Autodesk Fusion 360 part; units mm, degrees
(part 2 of 2)
  spline S14 degree 5 poles (-13.964533, 25.2) (-13.962061, 24.966553) (-13.956383, 24.502635) (-13.94566, 23.815681) (-13.926878, 22.917891) (-13.895401, 21.828032) (-13.855137, 20.773732) (-13.80525, 19.758375) (-13.745091, 18.78459) (-13.674758, 17.851981) (-13.594892, 16.957952) (-13.523933, 16.271322) (-13.466984, 15.771448) (-13.427386, 15.444802) (-13.407179, 15.28313) knots 0 0 0 0 0 0 0.1 0.2 0.3 0.4 0.5 0.6 0.7 0.8 0.9 1 1 1 1 1 1
  spline S15 degree 5 poles (-13.407179, 15.28313) (-13.396137, 15.263359) (-13.378996, 15.22331) (-13.368109, 15.161714) (-13.383287, 15.076541) (-13.451281, 14.964449) (-13.566539, 14.845147) (-13.725152, 14.715443) (-13.922038, 14.571096) (-14.152128, 14.407493) (-14.411349, 14.220248) (-14.697981, 14.00591) (-15.0128, 13.762359) (-15.357694, 13.488824) (-15.73468, 13.186004) (-16.144739, 12.856162) (-16.586746, 12.503236) (-17.056304, 12.132966) (-17.54468, 11.753005) (-18.03747, 11.373112) (-18.516745, 11.004243) (-18.963466, 10.657557) (-19.359795, 10.343456) (-19.691437, 10.070608) (-19.950048, 9.844948) (-20.135514, 9.668721) (-20.258658, 9.539357) (-20.342872, 9.448765) (-20.41611, 9.386384) (-20.504485, 9.341635) (-20.623844, 9.307073) (-20.78081, 9.278288) (-20.976661, 9.252807) (-21.210563, 9.229259) (-21.482071, 9.206674) (-21.790708, 9.184492) (-22.067067, 9.166839) (-22.290806, 9.15361) (-22.447275, 9.144795) (-22.527337, 9.140389) knots 0 0 0 0 0 0 0.02857143 0.05714286 0.08571429 0.11428571 0.14285714 0.17142857 0.2 0.22857143 0.25714286 0.28571429 0.31428571 0.34285714 0.37142857 0.4 0.42857143 0.45714286 0.48571429 0.51428571 0.54285714 0.57142857 0.6 0.62857143 0.65714286 0.68571429 0.71428571 0.74285714 0.77142857 0.8 0.82857143 0.85714286 0.88571429 0.91428571 0.94285714 0.97142857 1 1 1 1 1 1
  spline S16 degree 5 poles (-22.527337, 9.140389) (-22.534782, 9.132257) (-22.551108, 9.119693) (-22.579895, 9.111944) (-22.626933, 9.123822) (-22.704194, 9.176034) (-22.81318, 9.266751) (-22.971739, 9.396826) (-23.195327, 9.565352) (-23.491204, 9.768427) (-23.851155, 9.997537) (-24.255113, 10.24102) (-24.676282, 10.485947) (-25.085787, 10.719892) (-25.45738, 10.932679) (-25.772439, 11.118288) (-26.024118, 11.276365) (-26.223686, 11.414734) (-26.399129, 11.548396) (-26.585024, 11.694604) (-26.814317, 11.868763) (-27.110137, 12.080424) (-27.475633, 12.328182) (-27.891521, 12.598759) (-28.3256, 12.872564) (-28.739447, 13.127746) (-29.096109, 13.344754) (-29.367661, 13.510891) (-29.542161, 13.624396) (-29.632469, 13.699901) (-29.679781, 13.770002) (-29.730096, 13.86743) (-29.810663, 14.006795) (-29.915111, 14.173854) (-30.022328, 14.343768) (-30.107951, 14.492643) (-30.162056, 14.615407) (-30.190972, 14.726246) (-30.207343, 14.846076) (-30.222219, 14.991915) (-30.24042, 15.171174) (-30.263532, 15.386409) (-30.290852, 15.637231) (-30.321406, 15.923867) (-30.354419, 16.247692) (-30.389152, 16.610252) (-30.424903, 17.012708) (-30.460944, 17.455117) (-30.496481, 17.935767) (-30.530614, 18.450516) (-30.562281, 18.992027) (-30.590316, 19.550497) (-30.613514, 20.114573) (-30.630694, 20.672199) (-30.640764, 21.211485) (-30.642783, 21.721575) (-30.636028, 22.193507) (-30.620056, 22.621096) (-30.594767, 23.001764) (-30.560482, 23.337543) (-30.517829, 23.633921) (-30.46762, 23.898494) (-30.410725, 24.139655) (-30.347958, 24.365361) (-30.279935, 24.581643) (-30.207018, 24.791997) (-30.144919, 24.956973) (-30.096257, 25.079107) (-30.062889, 25.15982) (-30.045972, 25.2) knots 0 0 0 0 0 0 0.01538462 0.03076923 0.04615385 0.06153846 0.07692308 0.09230769 0.10769231 0.12307692 0.13846154 0.15384615 0.16923077 0.18461538 0.2 0.21538462 0.23076923 0.24615385 0.26153846 0.27692308 0.29230769 0.30769231 0.32307692 0.33846154 0.35384615 0.36923077 0.38461538 0.4 0.41538462 0.43076923 0.44615385 0.46153846 0.47692308 0.49230769 0.50769231 0.52307692 0.53846154 0.55384615 0.56923077 0.58461538 0.6 0.61538462 0.63076923 0.64615385 0.66153846 0.67692308 0.69230769 0.70769231 0.72307692 0.73846154 0.75384615 0.76923077 0.78461538 0.8 0.81538462 0.83076923 0.84615385 0.86153846 0.87692308 0.89230769 0.90769231 0.92307692 0.93846154 0.95384615 0.96923077 0.98461538 1 1 1 1 1 1
  spline S17 degree 5 poles (-35.799999, 25.2) (-35.857716, 25.156712) (-35.97592, 25.068059) (-36.161536, 24.928847) (-36.425914, 24.730563) (-36.786328, 24.460253) (-37.178908, 24.165818) (-37.605546, 23.845839) (-38.06599, 23.500506) (-38.557778, 23.131666) (-39.078002, 22.741497) (-39.514822, 22.413883) (-39.853268, 22.160048) (-40.083634, 21.987274) (-40.2, 21.9) knots 0 0 0 0 0 0 0.1 0.2 0.3 0.4 0.5 0.6 0.7 0.8 0.9 1 1 1 1 1 1
  spline S18 degree 5 poles (-7.251685, 9.474688) (-7.316766, 9.512048) (-7.450091, 9.589871) (-7.660018, 9.71659) (-7.959502, 9.906733) (-8.357963, 10.176766) (-8.767002, 10.471566) (-9.170812, 10.780262) (-9.554132, 11.090061) (-9.904845, 11.387591) (-10.217116, 11.660275) (-10.492886, 11.897621) (-10.739118, 12.09218) (-10.96578, 12.240707) (-11.183637, 12.344934) (-11.401893, 12.413255) (-11.626685, 12.459399) (-11.860987, 12.495777) (-12.104321, 12.528522) (-12.35221, 12.550684) (-12.59883, 12.547293) (-12.840058, 12.502059) (-13.076714, 12.403991) (-13.316787, 12.252645) (-13.5718, 12.05426) (-13.853764, 11.818935) (-14.172187, 11.557638) (-14.530366, 11.278714) (-14.92494, 10.987016) (-15.348078, 10.685204) (-15.788916, 10.374414) (-16.23528, 10.055179) (-16.67533, 9.728263) (-17.099141, 9.395474) (-17.500548, 9.060643) (-17.878143, 8.730033) (-18.23344, 8.410834) (-18.569489, 8.109951) (-18.889355, 7.832721) (-19.194554, 7.581563) (-19.483748, 7.354873) (-19.750714, 7.145276) (-19.985619, 6.940757) (-20.178259, 6.727494) (-20.32065, 6.492138) (-20.409985, 6.224389) (-20.451164, 5.919245) (-20.454223, 5.575435) (-20.432003, 5.194029) (-20.397764, 4.776997) (-20.362746, 4.325755) (-20.333949, 3.839836) (-20.314916, 3.317711) (-20.306339, 2.757479) (-20.306734, 2.157595) (-20.313084, 1.517597) (-20.321495, 0.838812) (-20.327855, 0.125116) (-20.328456, -0.616433) (-20.32074, -1.374637) (-20.303356, -2.134916) (-20.275945, -2.880746) (-20.239009, -3.594886) (-20.193751, -4.260684) (-20.141925, -4.86336) (-20.085669, -5.391269) (-20.027396, -5.837255) (-19.969528, -6.199769) (-19.914629, -6.484576) (-19.863943, -6.704252) (-19.814039, -6.875712) (-19.754645, -7.018248) (-19.664373, -7.151443) (-19.519774, -7.292529) (-19.3074, -7.453568) (-19.035103, -7.638642) (-18.724726, -7.845502) (-18.404345, -8.067303) (-18.100648, -8.294303) (-17.831346, -8.515571) (-17.597303, -8.720715) (-17.387506, -8.901628) (-17.184613, -9.054424) (-16.969919, -9.180947) (-16.729466, -9.291328) (-16.455457, -9.402009) (-16.14484, -9.530988) (-15.798752, -9.69393) (-15.421602, -9.899874) (-15.020326, -10.14724) (-14.603987, -10.426642) (-14.183416, -10.723577) (-13.770811, -11.021141) (-13.379401, -11.302783) (-13.022974, -11.554912) (-12.715738, -11.769892) (-12.471165, -11.94789) (-12.295635, -12.093535) (-12.183275, -12.213403) (-12.10937, -12.312955) (-12.026929, -12.394313) (-11.893759, -12.460455) (-11.701593, -12.520264) (-11.466708, -12.582483) (-11.21561, -12.64913) (-10.970951, -12.706907) (-10.746908, -12.732716) (-10.548658, -12.703423) (-10.36984, -12.605287) (-10.192728, -12.440298) (-9.995867, -12.219618) (-9.759968, -11.95953) (-9.475708, -11.675797) (-9.146515, -11.38075) (-8.783663, -11.084023) (-8.403132, -10.792461) (-8.021772, -10.510367) (-7.653742, -10.2396) (-7.306873, -9.979739) (-6.978942, -9.728205) (-6.660942, -9.481173) (-6.340562, -9.2345) (-6.005554, -8.984635) (-5.647219, -8.729565) (-5.263667, -8.469681) (-4.863667, -8.20886) (-4.463558, -7.952911) (-4.083315, -7.707674) (-3.743007, -7.477316) (-3.458888, -7.262376) (-3.240113, -7.058316) (-3.083992, -6.852825) (-2.978531, -6.629482) (-2.908356, -6.374567) (-2.859179, -6.082202) (-2.823813, -5.761836) (-2.800997, -5.433319) (-2.792171, -5.118206) (-2.799067, -4.832786) (-2.820648, -4.579328) (-2.851306, -4.341342) (-2.883618, -4.0939) (-2.910261, -3.811109) (-2.926583, -3.475921) (-2.931806, -3.084898) (-2.927712, -2.643652) (-2.917854, -2.164229) (-2.906556, -1.661705) (-2.898016, -1.151167) (-2.895328, -0.644408) (-2.89965, -0.147098) (-2.91081, 0.33966) (-2.927794, 0.8181) (-2.94928, 1.292445) (-2.974165, 1.767598) (-3.002065, 2.247839) (-3.033886, 2.735473) (-3.072209, 3.229633) (-3.120043, 3.726674) (-3.179682, 4.220423) (-3.251569, 4.702502) (-3.333056, 5.162573) (-3.417441, 5.588728) (-3.492333, 5.967551) (-3.539956, 6.285114) (-3.546166, 6.532117) (-3.508324, 6.708507) (-3.443506, 6.828224) (-3.396959, 6.924142) (-3.417583, 7.032207) (-3.528131, 7.172298) (-3.728551, 7.349665) (-4.004839, 7.559861) (-4.336561, 7.792682) (-4.700817, 8.034984) (-5.07472, 8.272853) (-5.438381, 8.493996) (-5.777747, 8.690093) (-6.087347, 8.859036) (-6.373518, 9.007565) (-6.650375, 9.148352) (-6.878149, 9.266932) (-7.059607, 9.365713) (-7.186605, 9.437328) (-7.251685, 9.474688) knots 0 0 0 0 0 0 0.00555556 0.01111111 0.01666667 0.02222222 0.02777778 0.03333333 0.03888889 0.04444444 0.05 0.05555556 0.06111111 0.06666667 0.07222222 0.07777778 0.08333333 0.08888889 0.09444444 0.1 0.10555556 0.11111111 0.11666667 0.12222222 0.12777778 0.13333333 0.13888889 0.14444444 0.15 0.15555556 0.16111111 0.16666667 0.17222222 0.17777778 0.18333333 0.18888889 0.19444444 0.2 0.20555556 0.21111111 0.21666667 0.22222222 0.22777778 0.23333333 0.23888889 0.24444444 0.25 0.25555556 0.26111111 0.26666667 0.27222222 0.27777778 0.28333333 0.28888889 0.29444444 0.3 0.30555556 0.31111111 0.31666667 0.32222222 0.32777778 0.33333333 0.33888889 0.34444444 0.35 0.35555556 0.36111111 0.36666667 0.37222222 0.37777778 0.38333333 0.38888889 0.39444444 0.4 0.40555556 0.41111111 0.41666667 0.42222222 0.42777778 0.43333333 0.43888889 0.44444444 0.45 0.45555556 0.46111111 0.46666667 0.47222222 0.47777778 0.48333333 0.48888889 0.49444444 0.5 0.50555556 0.51111111 0.51666667 0.52222222 0.52777778 0.53333333 0.53888889 0.54444444 0.55 0.55555556 0.56111111 0.56666667 0.57222222 0.57777778 0.58333333 0.58888889 0.59444444 0.6 0.60555556 0.61111111 0.61666667 0.62222222 0.62777778 0.63333333 0.63888889 0.64444444 0.65 0.65555556 0.66111111 0.66666667 0.67222222 0.67777778 0.68333333 0.68888889 0.69444444 0.7 0.70555556 0.71111111 0.71666667 0.72222222 0.72777778 0.73333333 0.73888889 0.74444444 0.75 0.75555556 0.76111111 0.76666667 0.77222222 0.77777778 0.78333333 0.78888889 0.79444444 0.8 0.80555556 0.81111111 0.81666667 0.82222222 0.82777778 0.83333333 0.83888889 0.84444444 0.85 0.85555556 0.86111111 0.86666667 0.87222222 0.87777778 0.88333333 0.88888889 0.89444444 0.9 0.90555556 0.91111111 0.91666667 0.92222222 0.92777778 0.93333333 0.93888889 0.94444444 0.95 0.95555556 0.96111111 0.96666667 0.97222222 0.97777778 0.98333333 0.98888889 0.99444444 1 1 1 1 1 1
  spline S19 degree 5 poles (-40.2, 19.435126) (-40.149452, 19.475964) (-40.050433, 19.557248) (-39.90661, 19.679254) (-39.715894, 19.84754) (-39.45302, 20.080899) (-39.140036, 20.348802) (-38.757974, 20.658525) (-38.300256, 21.011032) (-37.779317, 21.398606) (-37.221446, 21.806837) (-36.660563, 22.217012) (-36.132306, 22.608372) (-35.66817, 22.960396) (-35.289205, 23.255135) (-35.000865, 23.479382) (-34.785015, 23.627257) (-34.600802, 23.701515) (-34.406555, 23.711913) (-34.177474, 23.67408) (-33.925053, 23.608363) (-33.678893, 23.532293) (-33.471011, 23.45449) (-33.315202, 23.364998) (-33.206102, 23.240272) (-33.13084, 23.05705) (-33.077901, 22.805252) (-33.038632, 22.486233) (-33.006473, 22.107557) (-32.977022, 21.679287) (-32.947783, 21.20898) (-32.917834, 20.701777) (-32.887369, 20.161779) (-32.857286, 19.593015) (-32.828762, 19.000557) (-32.802816, 18.391626) (-32.77992, 17.776578) (-32.759479, 17.170267) (-32.740527, 16.589966) (-32.722642, 16.052706) (-32.706758, 15.572869) (-32.696067, 15.159571) (-32.696785, 14.814357) (-32.719215, 14.52823) (-32.777947, 14.280597) (-32.888646, 14.045885) (-33.065548, 13.79857) (-33.318253, 13.519712) (-33.650341, 13.19967) (-34.060347, 12.835846) (-34.542172, 12.431643) (-35.085703, 11.994925) (-35.677365, 11.53671) (-36.300666, 11.069741) (-36.9368, 10.607157) (-37.565091, 10.160997) (-38.164786, 9.742087) (-38.717072, 9.360165) (-39.207029, 9.023924) (-39.625577, 8.741082) (-39.971514, 8.518453) (-40.253317, 8.361985) (-40.491538, 8.276892) (-40.719461, 8.267505) (-40.972438, 8.335263) (-41.279562, 8.477169) (-41.652281, 8.683495) (-42.084145, 8.938436) (-42.557315, 9.222597) (-43.047002, 9.514916) (-43.526844, 9.794827) (-43.973667, 10.044313) (-44.373023, 10.250016) (-44.722915, 10.405286) (-45.027713, 10.511049) (-45.29243, 10.577355) (-45.518322, 10.623569) (-45.694416, 10.681773) (-45.804122, 10.78881) (-45.844251, 10.969039) (-45.845228, 11.216244) (-45.853969, 11.503616) (-45.911134, 11.798584) (-46.026094, 12.077954) (-46.166729, 12.336357) (-46.285066, 12.578038) (-46.33346, 12.812615) (-46.288743, 13.048324) (-46.157014, 13.289872) (-45.958752, 13.540504) (-45.719672, 13.802887) (-45.457716, 14.080729) (-45.182743, 14.378226) (-44.898955, 14.699075) (-44.606456, 15.045586) (-44.303104, 15.417839) (-43.98639, 15.812619) (-43.6548, 16.223111) (-43.307859, 16.640261) (-42.946478, 17.053795) (-42.573146, 17.453358) (-42.192258, 17.829642) (-41.810232, 18.175429) (-41.436098, 18.486876) (-41.080382, 18.763926) (-40.752269, 19.009826) (-40.516234, 19.186679) (-40.35372, 19.312218) (-40.250548, 19.394287) (-40.2, 19.435126) knots 0 0 0 0 0 0 0.00952381 0.01904762 0.02857143 0.03809524 0.04761905 0.05714286 0.06666667 0.07619048 0.08571429 0.0952381 0.1047619 0.11428571 0.12380952 0.13333333 0.14285714 0.15238095 0.16190476 0.17142857 0.18095238 0.19047619 0.2 0.20952381 0.21904762 0.22857143 0.23809524 0.24761905 0.25714286 0.26666667 0.27619048 0.28571429 0.2952381 0.3047619 0.31428571 0.32380952 0.33333333 0.34285714 0.35238095 0.36190476 0.37142857 0.38095238 0.39047619 0.4 0.40952381 0.41904762 0.42857143 0.43809524 0.44761905 0.45714286 0.46666667 0.47619048 0.48571429 0.4952381 0.5047619 0.51428571 0.52380952 0.53333333 0.54285714 0.55238095 0.56190476 0.57142857 0.58095238 0.59047619 0.6 0.60952381 0.61904762 0.62857143 0.63809524 0.64761905 0.65714286 0.66666667 0.67619048 0.68571429 0.6952381 0.7047619 0.71428571 0.72380952 0.73333333 0.74285714 0.75238095 0.76190476 0.77142857 0.78095238 0.79047619 0.8 0.80952381 0.81904762 0.82857143 0.83809524 0.84761905 0.85714286 0.86666667 0.87619048 0.88571429 0.8952381 0.9047619 0.91428571 0.92380952 0.93333333 0.94285714 0.95238095 0.96190476 0.97142857 0.98095238 0.99047619 1 1 1 1 1 1
  spline S20 degree 5 poles (-25.899999, 8.672189) (-25.984967, 8.74716) (-26.163615, 8.903833) (-26.460575, 9.159317) (-26.917421, 9.535675) (-27.566758, 10.03169) (-28.25241, 10.509223) (-28.925575, 10.925027) (-29.542266, 11.24726) (-30.075525, 11.466789) (-30.526083, 11.606509) (-30.911171, 11.699953) (-31.255466, 11.773808) (-31.579781, 11.825031) (-31.895023, 11.811855) (-32.211094, 11.685432) (-32.545508, 11.420383) (-32.925396, 11.028346) (-33.37816, 10.541477) (-33.924494, 10.002998) (-34.571372, 9.455734) (-35.302759, 8.929437) (-36.081114, 8.437585) (-36.857417, 7.982097) (-37.578688, 7.55571) (-38.196575, 7.145326) (-38.67539, 6.734917) (-39.000619, 6.308657) (-39.186593, 5.853855) (-39.26584, 5.360897) (-39.278928, 4.8233) (-39.264496, 4.237707) (-39.248251, 3.60395) (-39.244058, 2.924627) (-39.256546, 2.204615) (-39.283184, 1.450614) (-39.316551, 0.670684) (-39.346575, -0.126239) (-39.362602, -0.930726) (-39.355112, -1.733057) (-39.317487, -2.523459) (-39.247817, -3.292325) (-39.150548, -4.030457) (-39.038561, -4.729256) (-38.934035, -5.381058) (-38.858986, -5.980591) (-38.826335, -6.5264) (-38.831444, -7.022161) (-38.841879, -7.478356) (-38.792684, -7.912832) (-38.611528, -8.345269) (-38.238271, -8.792798) (-37.650221, -9.264428) (-36.873618, -9.758393) (-35.965893, -10.26574) (-35.003777, -10.772656) (-34.069131, -11.263294) (-33.23569, -11.722397) (-32.555565, -12.137967) (-32.045476, -12.504021) (-31.674082, -12.823009) (-31.381591, -13.098051) (-31.098054, -13.325654) (-30.762469, -13.48798) (-30.340663, -13.546053) (-29.81948, -13.455969) (-29.202007, -13.183446) (-28.50224, -12.720519) (-27.740512, -12.096905) (-26.941768, -11.366592) (-26.13348, -10.597787) (-25.343687, -9.861447) (-24.599028, -9.220712) (-23.922673, -8.719248) (-23.33253, -8.371703) (-22.838755, -8.14906) (-22.444231, -7.98563) (-22.147066, -7.800734) (-21.942329, -7.514785) (-21.824462, -7.070518) (-21.787311, -6.435873) (-21.823287, -5.600145) (-21.922795, -4.572297) (-22.073564, -3.378378) (-22.259991, -2.059361) (-22.462531, -0.668758) (-22.656931, 0.729526) (-22.81829, 2.067922) (-22.925294, 3.28206) (-22.964379, 4.317582) (-22.933943, 5.136993) (-22.848517, 5.72647) (-22.743027, 6.102802) (-22.676867, 6.320056) (-22.738697, 6.477159) (-22.991523, 6.666298) (-23.409009, 6.91383) (-23.910128, 7.20159) (-24.402242, 7.49497) (-24.820495, 7.768153) (-25.170523, 8.03164) (-25.435255, 8.259115) (-25.653808, 8.454009) (-25.815032, 8.597218) (-25.899999, 8.672189) knots 0 0 0 0 0 0 0.01 0.02 0.03 0.04 0.05 0.06 0.07 0.08 0.09 0.1 0.11 0.12 0.13 0.14 0.15 0.16 0.17 0.18 0.19 0.2 0.21 0.22 0.23 0.24 0.25 0.26 0.27 0.28 0.29 0.3 0.31 0.32 0.33 0.34 0.35 0.36 0.37 0.38 0.39 0.4 0.41 0.42 0.43 0.44 0.45 0.46 0.47 0.48 0.49 0.5 0.51 0.52 0.53 0.54 0.55 0.56 0.57 0.58 0.59 0.6 0.61 0.62 0.63 0.64 0.65 0.66 0.67 0.68 0.69 0.7 0.71 0.72 0.73 0.74 0.75 0.76 0.77 0.78 0.79 0.8 0.81 0.82 0.83 0.84 0.85 0.86 0.87 0.88 0.89 0.9 0.91 0.92 0.93 0.94 0.95 0.96 0.97 0.98 0.99 1 1 1 1 1 1
  spline S21 degree 5 poles (-40.2, -20.1) (-40.070612, -20.209158) (-39.809468, -20.426678) (-39.410646, -20.75057) (-38.864612, -21.177628) (-38.158809, -21.702993) (-37.431912, -22.218709) (-36.688764, -22.722538) (-35.937943, -23.210877) (-35.192901, -23.678421) (-34.473143, -24.117835) (-33.805518, -24.519395) (-33.225443, -24.870664) (-32.767007, -25.158828) (-32.453444, -25.37297) (-32.286721, -25.506553) (-32.23817, -25.559708) (-32.234886, -25.542486) (-32.185469, -25.4699) (-32.019779, -25.354344) (-31.700441, -25.203121) (-31.307891, -25.056873) (-30.934535, -24.933669) (-30.650671, -24.845553) (-30.499999, -24.799999) knots 0 0 0 0 0 0 0.05 0.1 0.15 0.2 0.25 0.3 0.35 0.4 0.45 0.5 0.55 0.6 0.65 0.7 0.75 0.8 0.85 0.9 0.95 1 1 1 1 1 1
  spline S22 degree 5 poles (-30.499999, -24.799999) (-30.496363, -24.810553) (-30.489336, -24.824863) (-30.479536, -24.825933) (-30.467947, -24.786539) (-30.456283, -24.672247) (-30.448444, -24.501505) (-30.445622, -24.286066) (-30.448807, -24.038807) (-30.458359, -23.771491) (-30.473636, -23.492751) (-30.493272, -23.208619) (-30.515425, -22.922913) (-30.538037, -22.637691) (-30.559089, -22.353651) (-30.576864, -22.070595) (-30.590156, -21.787729) (-30.59838, -21.503725) (-30.601688, -21.216835) (-30.601114, -20.924976) (-30.598652, -20.625847) (-30.597484, -20.316982) (-30.601631, -19.996067) (-30.615192, -19.661442) (-30.641708, -19.312552) (-30.683488, -18.950418) (-30.740915, -18.578115) (-30.811825, -18.201206) (-30.890695, -17.828319) (-30.970027, -17.46999) (-31.041981, -17.137319) (-31.099877, -16.840697) (-31.139863, -16.588482) (-31.162244, -16.385762) (-31.173636, -16.232892) (-31.186273, -16.124854) (-31.213971, -16.051863) (-31.268676, -15.999345) (-31.357547, -15.948968) (-31.484182, -15.882967) (-31.649256, -15.788686) (-31.85132, -15.661158) (-32.087333, -15.5007) (-32.353268, -15.311559) (-32.644698, -15.100095) (-32.957345, -14.873275) (-33.287768, -14.636761) (-33.633355, -14.394606) (-33.991973, -14.149698) (-34.361733, -13.903964) (-34.740702, -13.65868) (-35.126646, -13.414728) (-35.516742, -13.172882) (-35.907335, -12.934065) (-36.293605, -12.699659) (-36.6695, -12.471667) (-37.028436, -12.252494) (-37.363856, -12.044791) (-37.669847, -11.851275) (-37.941724, -11.67456) (-38.176649, -11.516983) (-38.374196, -11.380435) (-38.537043, -11.26618) (-38.670743, -11.174667) (-38.783391, -11.105292) (-38.88526, -11.056234) (-38.988633, -11.024128) (-39.106174, -11.004834) (-39.249186, -10.994346) (-39.425538, -10.98982) (-39.639816, -10.989593) (-39.843417, -10.992171) (-40.014544, -10.995531) (-40.136817, -10.998405) (-40.2, -11) knots 0 0 0 0 0 0 0.01428571 0.02857143 0.04285714 0.05714286 0.07142857 0.08571429 0.1 0.11428571 0.12857143 0.14285714 0.15714286 0.17142857 0.18571429 0.2 0.21428571 0.22857143 0.24285714 0.25714286 0.27142857 0.28571429 0.3 0.31428571 0.32857143 0.34285714 0.35714286 0.37142857 0.38571429 0.4 0.41428571 0.42857143 0.44285714 0.45714286 0.47142857 0.48571429 0.5 0.51428571 0.52857143 0.54285714 0.55714286 0.57142857 0.58571429 0.6 0.61428571 0.62857143 0.64285714 0.65714286 0.67142857 0.68571429 0.7 0.71428571 0.72857143 0.74285714 0.75714286 0.77142857 0.78571429 0.8 0.81428571 0.82857143 0.84285714 0.85714286 0.87142857 0.88571429 0.9 0.91428571 0.92857143 0.94285714 0.95714286 0.97142857 0.98571429 1 1 1 1 1 1
  spline S23 degree 5 poles (-11.380651, -26) (-11.388197, -25.910531) (-11.402672, -25.729202) (-11.42253, -25.450032) (-11.4453, -25.063451) (-11.467642, -24.556505) (-11.484034, -24.026467) (-11.494825, -23.474601) (-11.500601, -22.903035) (-11.50224, -22.314961) (-11.500981, -21.714879) (-11.498465, -21.108764) (-11.496844, -20.50441) (-11.498573, -19.910978) (-11.506026, -19.338129) (-11.521172, -18.795284) (-11.545217, -18.290819) (-11.578289, -17.831324) (-11.619018, -17.420756) (-11.664382, -17.059808) (-11.708878, -16.744756) (-11.746267, -16.468293) (-11.773521, -16.2221) (-11.794289, -15.998968) (-11.822268, -15.795034) (-11.885346, -15.612138) (-12.008974, -15.453868) (-12.202281, -15.322068) (-12.436677, -15.211941) (-12.655365, -15.113032) (-12.807341, -15.014838) (-12.872431, -14.910788) (-12.894793, -14.803655) (-12.948597, -14.699618) (-13.085321, -14.598945) (-13.316329, -14.493704) (-13.630512, -14.372693) (-14.00283, -14.224447) (-14.406896, -14.041175) (-14.82479, -13.821876) (-15.245145, -13.57058) (-15.661923, -13.294932) (-16.072933, -13.004628) (-16.478486, -12.709952) (-16.879942, -12.420194) (-17.278408, -12.142302) (-17.673128, -11.878965) (-18.061057, -11.629007) (-18.437276, -11.389401) (-18.79514, -11.156842) (-19.12658, -10.929434) (-19.42223, -10.708472) (-19.671888, -10.499853) (-19.864159, -10.31653) (-19.992077, -10.17283) (-20.059672, -10.07726) (-20.088653, -10.025604) (-20.123697, -9.99475) (-20.20687, -9.965518) (-20.360619, -9.934565) (-20.587881, -9.904642) (-20.867698, -9.877931) (-21.165433, -9.855989) (-21.445652, -9.841994) (-21.682682, -9.841809) (-21.875535, -9.866327) (-22.047955, -9.930248) (-22.232328, -10.047134) (-22.458111, -10.225525) (-22.73781, -10.464391) (-23.070333, -10.755311) (-23.444808, -11.084891) (-23.844265, -11.437111) (-24.249328, -11.795669) (-24.642002, -12.146396) (-25.00918, -12.479475) (-25.346902, -12.79219) (-25.65865, -13.087433) (-25.952489, -13.371396) (-26.238623, -13.651554) (-26.526755, -13.934505) (-26.823591, -14.223923) (-27.130139, -14.51833) (-27.43948, -14.809343) (-27.739693, -15.085552) (-28.016403, -15.335951) (-28.255518, -15.553654) (-28.44577, -15.739223) (-28.581625, -15.904811) (-28.665167, -16.075951) (-28.703251, -16.281648) (-28.705453, -16.546942) (-28.681386, -16.882643) (-28.639737, -17.284454) (-28.588384, -17.738354) (-28.5342, -18.22416) (-28.482988, -18.71979) (-28.439357, -19.205323) (-28.406625, -19.666927) (-28.386697, -20.101413) (-28.380163, -20.513882) (-28.386422, -20.914412) (-28.4038, -21.315132) (-28.429665, -21.727049) (-28.460556, -22.15718) (-28.492269, -22.605063) (-28.520075, -23.061079) (-28.539302, -23.510345) (-28.545878, -23.935672) (-28.536863, -24.320827) (-28.511027, -24.653815) (-28.469322, -24.929797) (-28.415629, -25.155094) (-28.355646, -25.343647) (-28.295371, -25.511762) (-28.239672, -25.673307) (-28.200687, -25.802721) (-28.174947, -25.900919) (-28.159341, -25.966889) (-28.151926, -26) knots 0 0 0 0 0 0 0.00869565 0.0173913 0.02608696 0.03478261 0.04347826 0.05217391 0.06086957 0.06956522 0.07826087 0.08695652 0.09565217 0.10434783 0.11304348 0.12173913 0.13043478 0.13913043 0.14782609 0.15652174 0.16521739 0.17391304 0.1826087 0.19130435 0.2 0.20869565 0.2173913 0.22608696 0.23478261 0.24347826 0.25217391 0.26086957 0.26956522 0.27826087 0.28695652 0.29565217 0.30434783 0.31304348 0.32173913 0.33043478 0.33913043 0.34782609 0.35652174 0.36521739 0.37391304 0.3826087 0.39130435 0.4 0.40869565 0.4173913 0.42608696 0.43478261 0.44347826 0.45217391 0.46086957 0.46956522 0.47826087 0.48695652 0.49565217 0.50434783 0.51304348 0.52173913 0.53043478 0.53913043 0.54782609 0.55652174 0.56521739 0.57391304 0.5826087 0.59130435 0.6 0.60869565 0.6173913 0.62608696 0.63478261 0.64347826 0.65217391 0.66086957 0.66956522 0.67826087 0.68695652 0.69565217 0.70434783 0.71304348 0.72173913 0.73043478 0.73913043 0.74782609 0.75652174 0.76521739 0.77391304 0.7826087 0.79130435 0.8 0.80869565 0.8173913 0.82608696 0.83478261 0.84347826 0.85217391 0.86086957 0.86956522 0.87826087 0.88695652 0.89565217 0.90434783 0.91304348 0.92173913 0.93043478 0.93913043 0.94782609 0.95652174 0.96521739 0.97391304 0.9826087 0.99130435 1 1 1 1 1 1
  spline S24 degree 5 poles (-35.499999, -26) (-35.583348, -25.95327) (-35.750996, -25.858269) (-36.005321, -25.71114) (-36.350223, -25.505562) (-36.791656, -25.231881) (-37.244241, -24.940117) (-37.708775, -24.628981) (-38.185476, -24.298115) (-38.673646, -23.948655) (-39.172323, -23.582159) (-39.578934, -23.276527) (-39.887924, -23.040764) (-40.095681, -22.880731) (-40.2, -22.799999) knots 0 0 0 0 0 0 0.1 0.2 0.3 0.4 0.5 0.6 0.7 0.8 0.9 1 1 1 1 1 1
  spline S25 degree 5 poles (14.045686, 25.2) (14.026679, 25.20986) (13.991231, 25.227461) (13.945749, 25.247506) (13.89915, 25.262651) (13.862026, 25.264318) (13.850846, 25.250684) (13.855566, 25.229938) (13.865264, 25.210855) (13.871751, 25.2) knots 0 0 0 0 0 0 0.2 0.4 0.6 0.8 1 1 1 1 1 1
  line L8 (14.10817, 25.167585) -> (13.983202, 25.232415)
  line L9 (13.858927, 25.221457) -> (13.884575, 25.178542)
  spline S26 degree 5 poles (21.4, 18.833166) (21.404845, 18.832018) (21.413971, 18.830201) (21.425972, 18.828916) (21.438361, 18.830282) (21.444879, 18.839631) (21.4384, 18.857077) (21.423658, 18.878584) (21.408736, 18.897264) (21.4, 18.907691) knots 0 0 0 0 0 0 0.2 0.4 0.6 0.8 1 1 1 1 1 1
  line L10 (21.44005, 18.859891) -> (21.35995, 18.955491)
  spline S27 degree 5 poles (21.4, 18.75) (21.3631, 18.792774) (21.288886, 18.877861) (21.176322, 19.004112) (21.023747, 19.169677) (20.828971, 19.372229) (20.630502, 19.571101) (20.429095, 19.767779) (20.226125, 19.964859) (20.022938, 20.165654) (19.820001, 20.373672) (19.616241, 20.59217) (19.407994, 20.8236) (19.189586, 21.069461) (18.954734, 21.330347) (18.697667, 21.605913) (18.414399, 21.894857) (18.103904, 22.194891) (17.767365, 22.503076) (17.407489, 22.816127) (17.027823, 23.130736) (16.63212, 23.443863) (16.223617, 23.753086) (15.804618, 24.05678) (15.376721, 24.353913) (14.940922, 24.643925) (14.586395, 24.87005) (14.317287, 25.036316) (14.136457, 25.145684) (14.045686, 25.2) knots 0 0 0 0 0 0 0.04 0.08 0.12 0.16 0.2 0.24 0.28 0.32 0.36 0.4 0.44 0.48 0.52 0.56 0.6 0.64 0.68 0.72 0.76 0.8 0.84 0.88 0.92 0.96 1 1 1 1 1 1
  line L11 (-40.2, -0.005933) -> (-9.4, -0.005933) construction
  line L12 (-9.4, -0.005933) -> (4.6, -0.005933) construction
  line L13 (-9.4, -0.005933) -> (-23.4, -0.005933) construction
  line L14 (4.6, -0.005933) -> (4.6, -6.005933) construction
  line L15 (-23.4, -0.005933) -> (-23.4, 5.994067) construction
  line L16 (19.4, -22) -> (19.4, 21.2)
  line L17 (17.4, 23.2) -> (-36.2, 23.2)
  line L18 (-38.2, 21.2) -> (-38.2, -22)
  line L19 (-36.2, -24) -> (17.4, -24)
  arc A23 (17.4, -24) -> (19.4, -22) centre (17.4, -22) ccw
  arc A24 (19.4, 21.2) -> (17.4, 23.2) centre (17.4, 21.2) ccw
  arc A25 (-36.2, 23.2) -> (-38.2, 21.2) centre (-36.2, 21.2) ccw
  arc A26 (-38.2, -22) -> (-36.2, -24) centre (-36.2, -22) ccw
  line L20 (4.6, -6.005933) -> (4.6, -8.255933)
  line L21 (-21.47495, 9.140389) -> (2.67495, 9.140389)
  line L22 (2.67495, 9.140389) -> (2.67495, -9.152255)
  line L23 (2.67495, -9.152255) -> (-21.47495, -9.152255)
  line L24 (-21.47495, -9.152255) -> (-21.47495, 9.140389)
  line L25 (-21.47495, 9.140389) -> (2.67495, -9.152255) construction
  line L26 (2.67495, 9.140389) -> (-21.47495, -9.152255) construction
  line L27 (-22.47495, 10.140389) -> (3.67495, 10.140389)
  line L28 (3.67495, 10.140389) -> (3.67495, -10.152255)
  line L29 (3.67495, -10.152255) -> (-22.47495, -10.152255)
  line L30 (-22.47495, -10.152255) -> (-22.47495, 10.140389)
  line L31 (2.67495, 9.140389) -> (-21.47495, 9.140389) construction
  line L32 (-21.47495, 9.140389) -> (-21.47495, -8.655649) construction
  line L33 (-21.47495, -8.655649) -> (2.67495, -8.655649) construction
  line L34 (2.67495, -8.655649) -> (2.67495, 9.140389) construction
  point P0 (7.05103, -15.07622)
  point P1 (6.833416, -14.831379)
  point P2 (5.8, -14)
  point P3 (5.004039, -13.246842)
  point P4 (3, -11.9)
  point P5 (2.193757, -11.255192)
  point P6 (0.684946, -10.141376)
  point P7 (-0.528509, -9.418997)
  point P8 (-1.303664, -9.37618)
  point P9 (-2.364881, -9.428861)
  point P10 (-2.833051, -9.537422)
  point P11 (-5.5, -11.6)
  point P12 (-8.6, -14.2)
  point P13 (-9.772693, -15.289634)
  point P14 (-9.847596, -15.465569)
  point P15 (-9.85, -15.9)
  point P16 (-9.9, -19.4)
  point P17 (-9.7, -23.999999)
  point P18 (19.8, -9.5)
  point P19 (18.3, -8.5)
  point P20 (18, -8.4)
  point P21 (16.7, -8.45)
  point P22 (16.268352, -8.47217)
  point P23 (16.073125, -8.568516)
  point P24 (13.8, -10.4)
  point P25 (10.9, -12.8)
  point P26 (9.4, -14.3)
  point P27 (19.156638, -6.650806)
  point P28 (18.8, -6.4)
  point P29 (18.7, -6.3)
  point P30 (18.55, -5.75)
  point P31 (18.2, -4.9)
  point P32 (18.3, -3.5)
  point P33 (18.5, -1.9)
  point P34 (18.5, 1.2)
  point P35 (18.3, 5.1)
  point P36 (18.3, 6.4)
  point P37 (18.1, 7.7)
  point P38 (18.1, 7.9)
  point P39 (18.9, 8.7)
  point P40 (19.8, 9.4)
  point P41 (13.5, -6.7)
  point P42 (11.8, -8.2)
  point P43 (11.235846, -8.970767)
  point P44 (9.7, -10.7)
  point P45 (8.9, -11.5)
  point P46 (7.1, -11.8)
  point P47 (6.951489, -11.717321)
  point P48 (6.717172, -11.544058)
  point P49 (6.177581, -11.202482)
  point P50 (5.256812, -10.530882)
  point P51 (3.2, -9)
  point P52 (1.1, -7.7)
  point P53 (-0.3, -6.9)
  point P54 (-0.423811, -6.834169)
  point P55 (-0.5, -6.65)
  point P56 (-1.1, -5.6)
  point P57 (-1.03, -5.44)
  point P58 (-1, -5.06)
  point P59 (-1.2, 0.8)
  point P60 (-1.4, 3.6)
  point P61 (-1.347097, 6.43103)
  point P62 (-1.25, 6.6)
  point P63 (-0.95, 7)
  point P64 (0.1, 8.2)
  point P65 (1.345563, 9.474688)
  point P66 (2.8, 10.4)
  point P67 (4.9, 11.6)
  point P68 (6.387176, 12.640055)
  point P69 (6.642448, 12.7645)
  point P70 (6.833901, 12.927236)
  point P71 (6.853047, 13.166553)
  point P72 (8.738865, 12.675155)
  point P73 (9.9, 11.8)
  point P74 (11.853178, 10.419089)
  point P75 (14.6, 8.6)
  point P76 (15.019467, 8.305909)
  point P77 (15.323938, 7.43489)
  point P78 (15.424144, 7.01865)
  point P79 (15.460001, 6.97)
  point P80 (15.470001, 6.82)
  point P81 (15.5, 5.3)
  point P82 (15.7, 1.7)
  point P83 (15.9, -1.6)
  point P84 (16, -4.7)
  point P85 (19, 12.5)
  point P86 (17.1, 10.8)
  point P87 (16.941283, 10.722166)
  point P88 (15.424153, 10.652981)
  point P89 (15.256132, 10.535456)
  point P90 (14.7, 10.9)
  point P91 (13, 12.2)
  point P92 (9.9, 14.1)
  point P93 (8.3, 15.2)
  point P94 (8.1, 15.6)
  point P95 (7.6, 16.4)
  point P96 (7.584244, 24.746012)
  point P97 (7.7, 24.999999)
  point P98 (11.1, 24.799999)
  point P99 (13.2, 23.499999)
  point P100 (15.3, 21.9)
  point P101 (19.768432, 17.823344)
  point P102 (-1.737306, 10.113739)
  point P103 (-2, 10)
  point P104 (-3.974541, 10.178663)
  point P105 (-4.5, 10.5)
  point P106 (-8.601278, 13.064444)
  point P107 (-11, 15)
  point P108 (-11.408835, 17.823344)
  point P109 (-11.841573, 24.855987)
  point P110 (-11.841573, 28.154907)
  point P111 (5.588692, 19.687321)
  point P112 (-13.784213, 19.446894)
  point P113 (-13.470829, 14.952984)
  point P114 (-14.3, 14.3)
  point P115 (-17.1, 12.1)
  point P116 (-20.1, 9.7)
  point P117 (-20.441762, 9.377297)
  point P118 (-20.923348, 9.260785)
  point P119 (-22.645343, 9.140389)
  point P120 (-23.249999, 9.6)
  point P121 (-25.899999, 11.2)
  point P122 (-26.999999, 12)
  point P123 (-29.499999, 13.6)
  point P124 (-29.7216, 13.849337)
  point P125 (-30.05902, 14.410315)
  point P126 (-30.199999, 14.8)
  point P127 (-30.27498, 15.491523)
  point P128 (-30.5, 18)
  point P129 (-30.615656, 22.648944)
  point P130 (-30.371506, 24.276613)
  point P131 (-37.399999, 23.999999)
  point P132 (-9.8, 11.3)
  point P133 (-11.1, 12.3)
  point P134 (-11.9, 12.5)
  point P135 (-12.8, 12.5)
  point P136 (-14, 11.7)
  point P137 (-16.99433, 9.474688)
  point P138 (-19.3, 7.5)
  point P139 (-20.3, 6.5)
  point P140 (-20.4, 4.8)
  point P141 (-20.327116, -0.09595)
  point P142 (-20, -6)
  point P143 (-19.8, -6.9)
  point P144 (-19.5, -7.3)
  point P145 (-18.1, -8.3)
  point P146 (-17.1, -9.1)
  point P147 (-15.8, -9.7)
  point P148 (-13.1, -11.5)
  point P149 (-12.2, -12.2)
  point P150 (-12, -12.4)
  point P151 (-11.4, -12.6)
  point P152 (-10.6, -12.7)
  point P153 (-9.845525, -12.056648)
  point P154 (-7.649659, -10.235404)
  point P155 (-5.6, -8.7)
  point P156 (-3.4, -7.2)
  point P157 (-2.9, -6.3)
  point P158 (-2.8, -4.9)
  point P159 (-2.9, -3.9)
  point P160 (-2.9, -1.2)
  point P161 (-3, 2.2)
  point P162 (-3.4, 5.5)
  point P163 (-3.5, 6.7)
  point P164 (-3.412768, 6.94432)
  point P165 (-3.8, 7.4)
  point P166 (-5.8, 8.7)
  point P167 (-38.699999, 20.7)
  point P168 (-35.099999, 23.399999)
  point P169 (-34.399999, 23.699999)
  point P170 (-33.599999, 23.499999)
  point P171 (-33.199999, 23.199999)
  point P172 (-32.999999, 22)
  point P173 (-32.799999, 18.3)
  point P174 (-32.699999, 14.9)
  point P175 (-32.999999, 13.9)
  point P176 (-36.399999, 11)
  point P177 (-40.2, 8.4)
  point P178 (-41.099999, 8.4)
  point P179 (-43.899999, 10)
  point P180 (-45.399999, 10.6)
  point P181 (-45.798736, 10.831704)
  point P182 (-45.899999, 11.7)
  point P183 (-46.299999, 12.7)
  point P184 (-45.899999, 13.6)
  point P185 (-44.399999, 15.3)
  point P186 (-41.999999, 18)
  point P187 (-29.475846, 11.2)
  point P188 (-31.171017, 11.752836)
  point P189 (-32.083801, 11.720237)
  point P190 (-34.219064, 9.76427)
  point P191 (-38.619989, 6.748822)
  point P192 (-39.271978, 4.743956)
  point P193 (-39.304577, 0.946122)
  point P194 (-39.15788, -3.943795)
  point P195 (-38.831885, -6.926644)
  point P196 (-38.326594, -8.654414)
  point P197 (-32.621692, -12.109955)
  point P198 (-31.099999, -13.3)
  point P199 (-29.299999, -13.2)
  point P200 (-23.699999, -8.6)
  point P201 (-22.1, -7.7)
  point P202 (-22.271119, -1.991553)
  point P203 (-22.750441, 6.073551)
  point P204 (-22.799999, 6.5)
  point P205 (-24.399999, 7.5)
  point P206 (-34.499999, -24.099999)
  point P207 (-32.299999, -25.499999)
  point P208 (-32.199999, -25.499999)
  point P209 (-30.470084, -24.778747)
  point P210 (-30.449999, -24.049999)
  point P211 (-30.550663, -22.462603)
  point P212 (-30.599999, -20.8)
  point P213 (-30.750984, -18.537976)
  point P214 (-31.150435, -16.483302)
  point P215 (-31.213157, -16.069526)
  point P216 (-31.449999, -15.9)
  point P217 (-32.75196, -15.02239)
  point P218 (-35.799999, -13)
  point P219 (-38.199999, -11.5)
  point P220 (-38.799999, -11.1)
  point P221 (-39.150148, -11.003144)
  point P222 (-11.5, -21.5)
  point P223 (-11.640677, -17.256563)
  point P224 (-11.796692, -15.999885)
  point P225 (-12.1, -15.4)
  point P226 (-12.8, -15)
  point P227 (-12.930808, -14.748883)
  point P228 (-13.973446, -14.231735)
  point P229 (-17.04714, -12.304942)
  point P230 (-19.457717, -10.674257)
  point P231 (-20.045764, -10.094551)
  point P232 (-20.119341, -10.004537)
  point P233 (-20.410001, -9.93)
  point P234 (-21.563329, -9.844355)
  point P235 (-22.252986, -10.069944)
  point P236 (-24.699999, -12.2)
  point P237 (-26.799999, -14.2)
  point P238 (-28.399999, -15.7)
  point P239 (-28.699999, -16.4)
  point P240 (-28.437387, -19.258645)
  point P241 (-28.452957, -22.050963)
  point P242 (-28.499999, -24.699999)
  point P243 (-28.299999, -25.499999)
  point P244 (-37.599999, -24.699999)
  point P245 (20.6, 19.6)
  point P246 (19.75, 20.45)
  point P247 (18.7, 21.6)
  point P248 (16.754692, 23.34487)
  point P249 (-9.4, -0.005933)
  dimension "d293" = 1
  dimension "d294" = 1
  dimension "d295" = 30.8
  dimension "d296" = 14
  dimension "d297" = 14
  dimension "d298" = 6
  dimension "d299" = 6
  dimension "d301" = 2
  dimension "d302" = 2.25
  dimension "d304" = -1
  dimension "d356" = 4.2
  text T0 "AGGRC\nTURTLE\nV3.2" font "Arial" height 4.2 align centre top in box 24.1499 x 17.796038 at (2.67495, 9.140389) x (-1, 0) y (0, -1) spacing 1 kerned
  constraint coincident L2 A9.end
  constraint tangent A5 A11
  constraint tangent A12 A13
  constraint coincident L2 A13.start
  constraint tangent A13 A16
  constraint coincident L2 S0.end
  constraint tangent A5 A17
  constraint tangent A10 A17
  constraint coincident L3 S2.start
  constraint coincident L3 S2.end
  constraint coincident L3 S10.start
  constraint tangent S12 A22
  constraint tangent S13 A22
  constraint coincident L7 S17.end
  constraint coincident L7 P177
  constraint coincident L7 S21.start
  constraint coincident L7 S22.end
  constraint coincident L5 S27.start
  constraint perpendicular L5 L11
  constraint parallel L11 L12
  constraint parallel L11 L13
  constraint perpendicular L12 L14
  constraint perpendicular L13 L15
  constraint tangent L19 A23
  constraint tangent L16 A23
  constraint tangent L16 A24
  constraint tangent L17 A24
  constraint equal A23 A24
  constraint tangent L17 A25
  constraint tangent L18 A25
  constraint equal A23 A25
  constraint tangent L18 A26
  constraint tangent L19 A26
  constraint equal A23 A26
  constraint parallel L14 L20
  constraint horizontal L21
  constraint perpendicular L21 L22
  constraint parallel L21 L23
  constraint parallel L22 L24
  constraint coincident S4
  constraint coincident L22
  measures "d293" radius of A17
  measures "d294" radius of A22
  measures "d301" radius of A23
extrude "Extrude33" cut sketch "Sketch24" sketch "Sketch24" against normal blind 0.7 contours S27 L16 L17 A24 | S10 S11 L16 L17 | S12 S13 A22 L17 L27 | S2 L16 | S14 S15 S16 L17 L27 L30 | A5 A6 A10 A11 A12 S1 A17 L16 | S18 L27 | S3 S4 S7 S8 S9 L27 L28 | S19 L17 L18 | A4 L16 L19 A23 | S20 L18 L30 | A13 A14 A15 A16 S0 L19 L29 | S18 L29 | S23 L19 L29 | S21 S22 L18 L19 picked at (17.56934, 22.778046) picked at (15.978956, 17.332254) picked at (-2.005446, 17.960188) picked at (19.08478, -0.065656) picked at (-20.056689, 18.457679) picked at (15.49268, -12.964271) picked at (-11.087971, 11.20776) picked at (7.753825, -0.331216) picked at (-34.659038, 19.665156) picked at (17.480153, -22.875563) picked at (-32.958317, -0.744098) picked at (0.005716, -17.170894) picked at (-12.168255, -11.201314) picked at (-18.23628, -17.700917) picked at (-36.113953, -16.255036) of sketch 2 text T0 bodies 2
chamfer "Chamfer21" distance 1 distance2 1 8 edges at (-7.895762, -25.2, 24.4) (-12.1, -25.2, 15.35) (-7.895762, -25.2, 6.3) (-3.691525, -25.2, 15.35) (-0.4, -25.2, 15.35) (3.801167, -25.2, 24.4) (8.002335, -25.2, 15.35) (3.801167, -25.2, 6.3) measured on face at (28.134112, -25.2, 18.6) measured on face at (28.134112, -25.2, 18.6) measured on face at (28.134112, -25.2, 18.6) measured on face at (28.134112, -25.2, 18.6) measured on face at (28.134112, -25.2, 18.6) measured on face at (28.134112, -25.2, 18.6) measured on face at (28.134112, -25.2, 18.6) measured on face at (28.134112, -25.2, 18.6) tangent chain off on bodies 1
chamfer "Chamfer22" distance 1 distance2 1 4 edges at (28.95, 26, 10.2) (33, 26, 8.25) (28.95, 26, 6.3) (24.899999, 26, 8.25) measured on face at (-4.633334, 26, 13.866667) measured on face at (-4.633334, 26, 13.866667) measured on face at (-4.633334, 26, 13.866667) measured on face at (-4.633334, 26, 13.866667) tangent chain off on bodies 1
chamfer "Chamfer23" distance 1 distance2 1 4 edges at (14.901509, -20.642423, 10) (-17.698491, -20.642423, 10) (15.255062, 19.91113, 10) (-17.910623, 19.769709, 10) measured on face at (16.750484, -19.883058, 10) measured on face at (-16.889047, -20.440086, 10) measured on face at (17.036708, 19.891568, 10) measured on face at (-16.878658, 19.67729, 10) tangent chain off on bodies 1
fillet "Fillet17" radius 2 16 edges at (-20.814214, -24.614214, 0) (-21.4, 0.4, 0) (-20.814214, 25.414214, 0) (9.4, 26, 0) (39.614214, 25.414214, 0) (40.2, 0.4, 0) (39.614214, -24.614214, 0) (9.4, -25.2, 0) (39.614214, -24.614214, 36.4) (40.2, 0.4, 36.4) (39.614214, 25.414214, 36.4) (9.4, 26, 36.4) (-20.814214, 25.414214, 36.4) (-21.4, 0.4, 36.4) (-20.814214, -24.614214, 36.4) (9.4, -25.2, 36.4) on bodies 1 2
chamfer "Chamfer20" distance 0.5 distance2 1 6 edges at (40.2, 0.4, 33.9) (40.2, 5.4, 32.65) (40.2, -4.6, 32.65) (-21.4, -4.6, 32.65) (-21.4, 0.4, 33.9) (-21.4, 5.4, 32.65) measured on face at (40.2, -17, 33.233467) measured on face at (40.2, -17, 33.233467) measured on face at (40.2, -17, 33.233467) measured on face at (-21.4, -17, 33.233467) measured on face at (-21.4, -17, 33.233467) measured on face at (-21.4, -17, 33.233467) tangent chain off on bodies 2
fillet "Fillet20" radius 2 2 edges at (22.47495, -10.140389, 36.05) (-3.67495, -10.140389, 36.05) on bodies 2
chamfer "Chamfer29" distance 5 distance2 1 4 edges at (9.4, 22.9, 34.4) (9.4, -22.1, 34.4) (-18.9, -22.1, 34.4) (37.7, -22.1, 34.4) measured on face at (-0.233333, 22.9, 32.4) measured on face at (0.166667, -22.1, 32.733333) measured on face at (-18.7, -22.1, 31.733333) measured on face at (37.5, -22.1, 31.733333) tangent chain off on bodies 2
chamfer "Chamfer30" distance 3 distance2 2 4 edges at (38.3, -22.7, 29.4) (38.3, 23.5, 29.4) (-19.5, 23.5, 29.4) (-19.5, -22.7, 29.4) measured on face at (18.633333, -22.9, 29.4) measured on face at (19.033333, 23.7, 29.4) measured on face at (19.033333, 23.7, 29.4) measured on face at (18.633333, -22.9, 29.4) tangent chain off on bodies 2
chamfer "Chamfer31" distance 8 angle 45 2 edges at (37.95, -10.6, 26.4) (-19.15, -17.6, 26.4) tangent chain off on bodies 2
chamfer "Chamfer32" distance 8 distance2 2.25 2 edges at (37.1, 2.9, 34.4) (-18.3, 0.4, 34.4) measured on face at (37.1, 1.066133, 31.733333) measured on face at (-18.3, -2.933867, 31.733333) tangent chain off on bodies 2
fillet "Fillet22" radius 0.4 4 edges at (38.8, 6.9, 26.4) (38.8, 5.9, 28.4) (-20, 4.4, 26.4) (-20, 3.4, 28.4) on bodies 2
fillet "Fillet23" radius 0.5 6 edges at (9.4, 24.1, 29.4) (9.4, -23.3, 29.4) (-18, -23.3, 30.4) (36.8, -23.3, 30.4) (36.8, 24.1, 30.4) (-18, 24.1, 30.4) on bodies 2
hidden bodies 2
named bodies: "Base", "Top"
